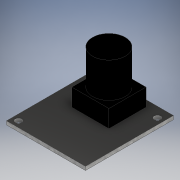
# Autodesk Inventor part: Pixy Sketch
Saved by Autodesk Inventor 2018 (Build 220112000, 112)
## iProperties
Created: 2018-08-30
Part Number: Pixy Sketch
Material: Generic
Document SubType Name: Modeling
Designer: matth
Density: 1 g/cm^3
Appearance: Default
Author: matth
Autodesk Inventor part; units mm, degrees
ref_plane "YZ Plane" through (0, 0, 0) normal (1, 0, 0) x (0, 1, 0)
ref_plane "XZ Plane" through (0, 0, 0) normal (0, 1, 0) x (-1, 0, 0)
ref_plane "XY Plane" through (0, 0, 0) normal (0, 0, 1) x (1, 0, 0)
sketch "Sketch1" plane through (0, 0, 0) normal (0, 0, 1) x (1, 0, 0)
  line L0 (0, 0) -> (0, 8.5)
  line L1 (0, 8.5) -> (8.5, 8.5)
  line L2 (8.5, 8.5) -> (8.5, -8.5)
  line L3 (8.5, -8.5) -> (-8.5, -8.5)
  line L4 (-8.5, -8.5) -> (-8.5, 8.5)
  line L5 (-8.5, 8.5) -> (0, 8.5)
  line L6 (0, 8.5) -> (0, 10.25)
  line L7 (0, 10.25) -> (-15.33, 10.25)
  line L8 (-15.33, 10.25) -> (-15.33, 6.92)
  circle A0 centre (-15.33, 6.92) radius 1.5
  line L9 (0, 10.25) -> (15.33, 10.25)
  line L10 (15.33, 10.25) -> (15.33, 6.92)
  circle A1 centre (15.33, 6.92) radius 1.5
  line L11 (-15.33, 6.92) -> (-15.33, -26.08)
  circle A2 centre (-15.33, -26.08) radius 1.5
  line L12 (0, 0) -> (0, 6.92)
  line L13 (-16.83, 6.92) -> (-18.08, 6.92)
  line L14 (-18.08, 6.92) -> (-18.08, -28.83)
  line L15 (-18.08, 6.92) -> (-18.08, 11.5)
  line L16 (-18.08, 11.5) -> (-3.5327, 11.5)
  line L17 (-3.5327, 11.5) -> (18.0803, 11.5)
  line L18 (18.0803, 11.5) -> (18.0803, -28.83)
  line L19 (18.0803, -28.83) -> (-18.08, -28.83)
  dimension "d8" = 3
  dimension "d0" = 8.5
  dimension "d1" = 8.5
  dimension "d2" = 17
  dimension "d3" = 17
  dimension "d4" = 17
  dimension "d5" = 1.75
  dimension "d6" = 15.33
  dimension "d7" = 3.33
  dimension "d9" = 15.33
  dimension "d10" = 3.33
  dimension "d11" = 3
  dimension "d12" = 33
  dimension "d13" = 3
  dimension "d14" = 1.25
  dimension "d15" = 35.75
  dimension "d16" = 4.58
  dimension "d17" = 21.613
  constraints: 40 end point, 10 perpendicular, 4 point on line, 4 vertical, 3 coincident, 2 centre point, 2 horizontal, 1 horizontal alignment, 2 other
  measures "d0" distance of L0.start L0.end
  measures "d1" distance of L0.end L1.end
  measures "d2" distance of L1.end L2.end
  measures "d3" distance of L2.end L3.end
  measures "d4" distance of L3.end L4.end
  measures "d5" distance of L0.end L6.end
  measures "d6" distance of L6.end L7.end
  measures "d7" distance of L7.end L8.end
  measures "d9" distance of L6.end L9.end
  measures "d10" distance of L9.end L10.end
  measures "d11" diameter of A1
  measures "d12" distance of L11.start L11.end
  measures "d13" diameter of A2
  measures "d14" distance of L13.start L13.end
  measures "d15" distance of L13.end L14.end
  measures "d16" distance of L13.end L15.end
  measures "d17" distance of L16.end L17.end
extrude "Extrusion1" add sketch "Sketch1" along normal blind 1.65
sketch "Sketch2" plane through (0, 0, 1.65) normal (0, 0, 1) x (1, 0, 0)
  line L0 (-8.5, 8.5) -> (-8.5, -8.5) projected
  line L1 (8.5, 8.5) -> (8.5, -8.5) projected
  line L2 (-8.5, 8.5) -> (8.5, 8.5)
  line L3 (8.5, 8.5) -> (8.5, -8.5)
  line L4 (8.5, -8.5) -> (-8.5, -8.5)
  line L5 (-8.5, -8.5) -> (-8.5, 8.5)
  point P0 (0, 0)
  constraints: 8 end point, 2 parallel, 1 horizontal, 1 perpendicular
extrude "Extrusion2" add sketch "Sketch2" along normal blind 8 and the other way blind 1.65
sketch "Sketch3" plane through (0, 0, 9.65) normal (0, 0, 1) x (1, 0, 0)
  circle A0 centre (0, 0) radius 7.5
  dimension "d24" = 15
  constraints: 1 centre point, 1 coincident
  measures "d24" diameter of A0
extrude "Extrusion3" add sketch "Sketch3" along normal blind 16
body "Solid1"
